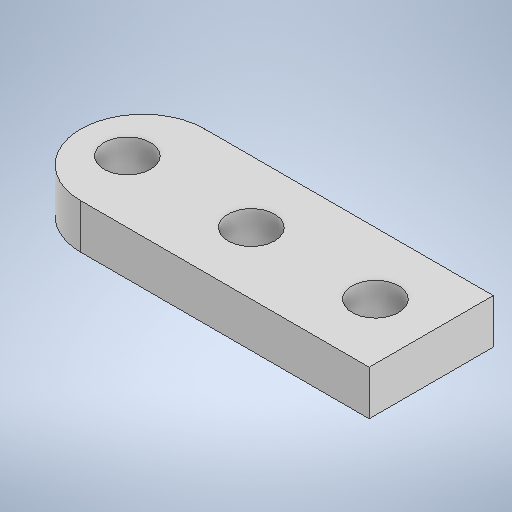
# Autodesk Inventor part: CH-1-03-RearGearboxSpacer_01
Saved by Autodesk Inventor 2025.1 (Build 291241020, 241B)
## iProperties
Created: 2024-10-23
Part Number: CH-1-03-RearGearboxSpacer_01
Material: Generic
Document SubType Name: Modeling
Designer: aidan
Density: 1 g/cm^3
Appearance: Default
Author: aidan
Autodesk Inventor part; units mm, degrees
ref_plane "YZ Plane" through (0, 0, 0) normal (1, 0, 0) x (0, 1, 0)
ref_plane "XZ Plane" through (0, 0, 0) normal (0, 1, 0) x (-1, 0, 0)
ref_plane "XY Plane" through (0, 0, 0) normal (0, 0, 1) x (1, 0, 0)
sketch "Sketch1" plane through (0, 0, 0) normal (1, 0, 0) x (0, 1, 0)
  line L0 (0, 0) -> (9.144, 0)
  line L1 (9.144, 0) -> (9.144, -25.4)
  line L2 (9.144, -25.4) -> (0, -25.4)
  line L3 (0, -25.4) -> (0, 0)
  dimension "d0" = 25.4
  dimension "d1" = 9.144
  constraints: 8 end point, 2 parallel, 1 horizontal, 1 perpendicular
  measures "d0" distance of L2.end L0.start
  measures "d1" distance of L1.end L2.end
extrude "Extrusion1" add sketch "Sketch1" along normal blind 63.5
sketch "Sketch2" plane through (0, 9.144, 0) normal (0, 1, 0) x (1, 0, 0)
  line L0 (0, 25.4) -> (0, 0) projected
  line L1 (0, 12.7) -> (6.35, 12.7)
  line L2 (6.35, 12.7) -> (31.75, 12.7)
  line L3 (31.75, 12.7) -> (57.15, 12.7)
  circle A0 centre (6.35, 12.7) radius 4.7625
  circle A1 centre (31.75, 12.7) radius 4.7625
  circle A2 centre (57.15, 12.7) radius 4.7625
  dimension "d4" = 6.35
  dimension "d5" = 25.4
  dimension "d6" = 25.4
  dimension "d7" = 9.525
  dimension "d8" = 9.525
  dimension "d9" = 9.525
  constraints: 6 end point, 3 centre point, 3 coincident, 2 point on line, 1 horizontal, 1 midpoint
  measures "d4" distance of L1.start L1.end
  measures "d5" distance of L1.end L2.end
  measures "d6" distance of L2.end L3.end
  measures "d7" diameter of A0
  measures "d8" diameter of A1
  measures "d9" diameter of A2
sketch "Sketch3" plane through (0, 0, 0) normal (-1, 0, 0) x (0, 0, 1)
  line L0 (-25.4, 0) -> (-25.4, 9.144) projected
  line L1 (0, 0) -> (-25.4, 0)
  line L2 (-25.4, 0) -> (-25.4, 9.144)
  line L3 (-25.4, 9.144) -> (0, 9.144)
  line L4 (0, 9.144) -> (0, 0)
  constraints: 8 end point, 2 parallel, 1 horizontal, 1 perpendicular
extrude "Extrusion2" add sketch "Sketch3" along normal blind 3.175
fillet "Fillet1" radius 12.7 2 edges at (-3.175, 4.572, -25.4) (-3.175, 4.572, 0)
extrude "Extrusion3" cut sketch "Sketch2" against normal blind 25.4
sketch "Sketch4" plane through (63.5, 0, 0) normal (1, 0, 0) x (0, 0, -1)
  line L0 (25.4, 0) -> (25.4, 9.144) projected
  line L1 (25.4, 9.144) -> (0, 9.144) projected
  line L2 (0, 9.144) -> (0, 0) projected
  line L3 (0, 0) -> (25.4, 0) projected
extrude "Extrusion4" add sketch "Sketch4" along normal blind 5.08
body "Solid1"
